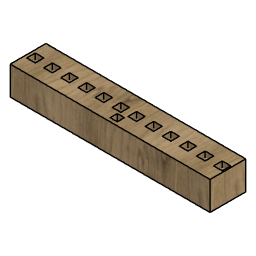
dissertation_demo2 v0 (Autodesk Fusion 360 design; units mm, degrees)
Autodesk Fusion 360 part; units mm, degrees
sketch "Sketch1" plane through (0, 0, 0) normal (0, 0, 1) x (1, 0, 0)
  line L0 (280, 50) -> (-280, 50)
  line L1 (-280, 50) -> (-280, -50)
  line L2 (-280, -50) -> (280, -50)
  line L3 (280, -50) -> (280, 50)
  line L4 (280, 50) -> (-280, -50) construction
  line L5 (-280, 50) -> (280, -50) construction
  dimension "d1" = 560
  dimension "d2" = 100
  constraint horizontal L0
  constraint perpendicular L0 L1
  constraint parallel L0 L2
  constraint parallel L1 L3
  constraint coincident L4 origin
  constraint coincident L5 origin
  measures "d1" distance of L1.end L2.end
  measures "d2" distance of L0.end L1.end
extrude "Extrude1" add sketch "Sketch1" along normal blind 50 makes body 1
sketch "Sketch2" plane through (0, 0, 50) normal (0, 0, 1) x (-1, 0, 0)
  line L0 (-280, 50) -> (-280, -50)
  line L1 (-280, -50) -> (280, -50)
  line L2 (280, -50) -> (280, 50)
  line L3 (280, 50) -> (-280, 50)
  line L4 (8, -12) -> (32, -12)
  line L5 (32, -12) -> (32, 12)
  line L6 (32, 12) -> (8, 12)
  line L7 (8, 12) -> (8, -12)
  dimension "d5" = 24
  dimension "d6" = 24
  constraint horizontal L4
  constraint vertical L5
  constraint horizontal L6
  constraint vertical L7
  measures "d5" distance of L4.start L4.end
  measures "d6" distance of L4.start L6.end
extrude "Extrude2" cut sketch "Sketch2" against normal blind 175 contours L4 L5 L6 L7 bodies 1
sketch "Sketch3" plane through (0, 0, 0) normal (0, 0, -1) x (1, 0, 0)
  line L0 (-8, -12) -> (-32, -12)
  line L1 (-32, -12) -> (-32, 12)
  line L2 (-32, 12) -> (-8, 12)
  line L3 (-8, 12) -> (-8, -12)
  line L4 (280, -50) -> (280, 50)
  line L5 (280, 50) -> (-280, 50)
  line L6 (-280, 50) -> (-280, -50)
  line L7 (-280, -50) -> (280, -50)
  line L8 (-275, 145) -> (275, 145)
  line L9 (275, 145) -> (275, -145)
  line L10 (275, -145) -> (-275, -145)
  line L11 (-275, -145) -> (-275, 145)
  line L12 (-275, 145) -> (275, -145) construction
  line L13 (275, 145) -> (-275, -145) construction
  dimension "d9" = 550
  dimension "d10" = 290
  constraint horizontal L8
  constraint perpendicular L8 L9
  constraint parallel L8 L10
  constraint parallel L9 L11
  constraint coincident L12 origin
  constraint coincident L13 origin
  measures "d9" distance of L9.end L10.end
  measures "d10" distance of L8.end L9.end
extrude "Extrude3" cut sketch "Sketch3" along normal blind 5 contours L7 L9 L10 L11 | L5 L7 L9 L11 | L5 L8 L9 L11 bodies 1
sketch "Sketch4" plane through (0, 0, 50) normal (0, 0, 1) x (-1, 0, 0)
  line L0 (32, -12) -> (8, -12)
  line L1 (8, -12) -> (8, 12)
  line L2 (8, 12) -> (32, 12)
  line L3 (32, 12) -> (32, -12)
  line L4 (-280, 50) -> (-280, -50)
  line L5 (-280, -50) -> (280, -50)
  line L6 (280, -50) -> (280, 50)
  line L7 (280, 50) -> (-280, 50)
sketch "Sketch5" plane through (0, 0, 50) normal (0, 0, 1) x (1, 0, 0)
  line L0 (36, 12) -> (12, 12)
  line L1 (12, 12) -> (12, -12)
  line L2 (12, -12) -> (36, -12)
  line L3 (36, -12) -> (36, 12)
  line L4 (36, 12) -> (12, -12) construction
  line L5 (12, 12) -> (36, -12) construction
  point P0 (24, 0)
  dimension "d13" = 24
  dimension "d14" = 24
  constraint horizontal L0
  constraint perpendicular L0 L1
  constraint parallel L0 L2
  constraint parallel L1 L3
  constraint coincident L4 P0
  constraint coincident L5 P0
  measures "d13" distance of L1.end L2.end
  measures "d14" distance of L0.end L1.end
extrude "Extrude4" cut sketch "Sketch5" against normal blind 30 bodies 1
sketch "Sketch6" plane through (0, 0, 0) normal (0, 0, 1) x (1, 0, 0)
  line L0 (-275, -45) -> (275, -45)
  line L1 (275, -45) -> (275, 45)
  line L2 (275, 45) -> (-275, 45)
  line L3 (-275, 45) -> (-275, -45)
  line L4 (-275, -45) -> (275, 45) construction
  line L5 (275, -45) -> (-275, 45) construction
  dimension "d17" = 550
  dimension "d18" = 90
  constraint horizontal L0
  constraint perpendicular L0 L1
  constraint parallel L0 L2
  constraint parallel L1 L3
  constraint coincident L4 origin
  constraint coincident L5 origin
  measures "d17" distance of L1.end L2.end
  measures "d18" distance of L0.end L1.end
extrude "Extrude5" cut sketch "Sketch6" along normal blind 30 bodies 1
sketch "Sketch7" plane through (0, 0, 50) normal (0, 0, 1) x (1, 0, 0)
  line L0 (-80, 12) -> (-56, 12)
  line L1 (-56, 12) -> (-56, -12)
  line L2 (-56, -12) -> (-80, -12)
  line L3 (-80, -12) -> (-80, 12)
  line L4 (-80, 12) -> (-56, -12) construction
  line L5 (-56, 12) -> (-80, -12) construction
  line L6 (-104, 12) -> (-128, -12) construction
  line L7 (-128, 12) -> (-104, 12)
  line L8 (-128, -12) -> (-128, 12)
  line L9 (-128, 12) -> (-104, -12) construction
  line L10 (-104, -12) -> (-128, -12)
  line L11 (-104, 12) -> (-104, -12)
  line L12 (-152, 12) -> (-176, -12) construction
  line L13 (-176, 12) -> (-152, 12)
  line L14 (-176, -12) -> (-176, 12)
  line L15 (-176, 12) -> (-152, -12) construction
  line L16 (-152, -12) -> (-176, -12)
  line L17 (-152, 12) -> (-152, -12)
  line L18 (-200, 12) -> (-224, -12) construction
  line L19 (-224, 12) -> (-200, 12)
  line L20 (-224, -12) -> (-224, 12)
  line L21 (-224, 12) -> (-200, -12) construction
  line L22 (-200, -12) -> (-224, -12)
  line L23 (-200, 12) -> (-200, -12)
  line L24 (-248, 12) -> (-272, -12) construction
  line L25 (-272, 12) -> (-248, 12)
  line L26 (-272, -12) -> (-272, 12)
  line L27 (-272, 12) -> (-248, -12) construction
  line L28 (-248, -12) -> (-272, -12)
  line L29 (-248, 12) -> (-248, -12)
  point P0 (-68, 0)
  dimension "d21" = 24
  dimension "d22" = 24
  dimension "d25" = -192
  dimension "d26" = 0
  constraint horizontal L0
  constraint perpendicular L0 L1
  constraint parallel L0 L2
  constraint parallel L1 L3
  constraint coincident L4 P0
  constraint coincident L5 P0
  measures "d21" distance of L1.end L2.end
  measures "d22" distance of L0.end L1.end
extrude "Extrude6" cut sketch "Sketch7" against normal blind 40 bodies 1
sketch "Sketch8" plane through (0, 0, 50) normal (0, 0, 1) x (-1, 0, 0)
  line L0 (224, 12) -> (224, -12)
  line L1 (224, -12) -> (200, -12)
  line L2 (200, -12) -> (200, 12)
  line L3 (200, 12) -> (224, 12)
  line L4 (176, 12) -> (176, -12)
  line L5 (176, -12) -> (152, -12)
  line L6 (152, -12) -> (152, 12)
  line L7 (152, 12) -> (176, 12)
  line L8 (272, 12) -> (272, -12)
  line L9 (272, -12) -> (248, -12)
  line L10 (248, -12) -> (248, 12)
  line L11 (248, 12) -> (272, 12)
  line L12 (128, 12) -> (128, -12)
  line L13 (128, -12) -> (104, -12)
  line L14 (104, -12) -> (104, 12)
  line L15 (104, 12) -> (128, 12)
  line L16 (56, -12) -> (56, 12)
  line L17 (56, 12) -> (80, 12)
  line L18 (80, 12) -> (80, -12)
  line L19 (80, -12) -> (56, -12)
  line L20 (-12, -12) -> (-36, -12)
  line L21 (-36, -12) -> (-36, 12)
  line L22 (-36, 12) -> (-12, 12)
  line L23 (-12, 12) -> (-12, -12)
  line L24 (32, -12) -> (8, -12)
  line L25 (8, -12) -> (8, 12)
  line L26 (8, 12) -> (32, 12)
  line L27 (32, 12) -> (32, -12)
  line L28 (-280, 50) -> (-280, -50)
  line L29 (-280, -50) -> (280, -50)
  line L30 (280, -50) -> (280, 50)
  line L31 (280, 50) -> (-280, 50)
  line L32 (-60, -12) -> (-84, -12)
  line L33 (-84, -12) -> (-84, 12)
  line L34 (-84, 12) -> (-60, 12)
  line L35 (-60, 12) -> (-60, -12)
  line L36 (-60, -12) -> (-84, 12) construction
  line L37 (-84, -12) -> (-60, 12) construction
  line L38 (-132, 12) -> (-108, 12)
  line L39 (-108, 12) -> (-108, -12)
  line L40 (-108, -12) -> (-132, -12)
  line L41 (-132, -12) -> (-108, 12) construction
  line L42 (-108, -12) -> (-132, 12) construction
  line L43 (-132, -12) -> (-132, 12)
  line L44 (-180, 12) -> (-156, 12)
  line L45 (-156, 12) -> (-156, -12)
  line L46 (-156, -12) -> (-180, -12)
  line L47 (-180, -12) -> (-156, 12) construction
  line L48 (-156, -12) -> (-180, 12) construction
  line L49 (-180, -12) -> (-180, 12)
  line L50 (-228, 12) -> (-204, 12)
  line L51 (-204, 12) -> (-204, -12)
  line L52 (-204, -12) -> (-228, -12)
  line L53 (-228, -12) -> (-204, 12) construction
  line L54 (-204, -12) -> (-228, 12) construction
  line L55 (-228, -12) -> (-228, 12)
  line L56 (-276, 12) -> (-252, 12)
  line L57 (-252, 12) -> (-252, -12)
  line L58 (-252, -12) -> (-276, -12)
  line L59 (-276, -12) -> (-252, 12) construction
  line L60 (-252, -12) -> (-276, 12) construction
  line L61 (-276, -12) -> (-276, 12)
  point P0 (-72, 0)
  point P1 (-120, 0)
  point P2 (-168, 0)
  point P3 (-216, 0)
  point P4 (-264, 0)
  dimension "d29" = 24
  dimension "d30" = 24
  dimension "d33" = -192
  dimension "d34" = 0
  constraint horizontal L32
  constraint perpendicular L32 L33
  constraint parallel L32 L34
  constraint parallel L33 L35
  constraint coincident L36 P0
  constraint coincident L37 P0
  measures "d29" distance of L33.end L34.end
  measures "d30" distance of L32.end L33.end
extrude "Extrude7" cut sketch "Sketch8" against normal blind 60 contours L32 L33 L34 L35 | L38 L39 L40 L43 | L44 L45 L46 L49 | L50 L51 L52 L55 | L56 L57 L58 L61 bodies 1
sketch "Sketch9" plane through (0, 0, 50) normal (0, 0, 1) x (-1, 0, 0)
  line L0 (-204, 12) -> (-204, -12)
  line L1 (-204, -12) -> (-228, -12)
  line L2 (-228, -12) -> (-228, 12)
  line L3 (-228, 12) -> (-204, 12)
  line L4 (-156, 12) -> (-156, -12)
  line L5 (-156, -12) -> (-180, -12)
  line L6 (-180, -12) -> (-180, 12)
  line L7 (-180, 12) -> (-156, 12)
  line L8 (-252, 12) -> (-252, -12)
  line L9 (-252, -12) -> (-276, -12)
  line L10 (-276, -12) -> (-276, 12)
  line L11 (-276, 12) -> (-252, 12)
  line L12 (-108, 12) -> (-108, -12)
  line L13 (-108, -12) -> (-132, -12)
  line L14 (-132, -12) -> (-132, 12)
  line L15 (-132, 12) -> (-108, 12)
  line L16 (-84, -12) -> (-84, 12)
  line L17 (-84, 12) -> (-60, 12)
  line L18 (-60, 12) -> (-60, -12)
  line L19 (-60, -12) -> (-84, -12)
  line L20 (224, 12) -> (224, -12)
  line L21 (224, -12) -> (200, -12)
  line L22 (200, -12) -> (200, 12)
  line L23 (200, 12) -> (224, 12)
  line L24 (176, 12) -> (176, -12)
  line L25 (176, -12) -> (152, -12)
  line L26 (152, -12) -> (152, 12)
  line L27 (152, 12) -> (176, 12)
  line L28 (272, 12) -> (272, -12)
  line L29 (272, -12) -> (248, -12)
  line L30 (248, -12) -> (248, 12)
  line L31 (248, 12) -> (272, 12)
  line L32 (128, 12) -> (128, -12)
  line L33 (128, -12) -> (104, -12)
  line L34 (104, -12) -> (104, 12)
  line L35 (104, 12) -> (128, 12)
  line L36 (56, -12) -> (56, 12)
  line L37 (56, 12) -> (80, 12)
  line L38 (80, 12) -> (80, -12)
  line L39 (80, -12) -> (56, -12)
  line L40 (-12, -12) -> (-36, -12)
  line L41 (-36, -12) -> (-36, 12)
  line L42 (-36, 12) -> (-12, 12)
  line L43 (-12, 12) -> (-12, -12)
  line L44 (32, -12) -> (8, -12)
  line L45 (8, -12) -> (8, 12)
  line L46 (8, 12) -> (32, 12)
  line L47 (32, 12) -> (32, -12)
  line L48 (-280, 50) -> (-280, -50)
  line L49 (-280, -50) -> (280, -50)
  line L50 (280, -50) -> (280, 50)
  line L51 (280, 50) -> (-280, 50)
  line L52 (10, 40) -> (-10, 40)
  line L53 (-10, 40) -> (-10, 20)
  line L54 (-10, 20) -> (10, 20)
  line L55 (10, 20) -> (10, 40)
  line L56 (10, 40) -> (-10, 20) construction
  line L57 (-10, 40) -> (10, 20) construction
  point P0 (0, 30)
  dimension "d37" = 20
  constraint horizontal L52
  constraint perpendicular L52 L53
  constraint parallel L52 L54
  constraint parallel L53 L55
  constraint coincident L56 P0
  constraint coincident L57 P0
  measures "d37" distance of L53.end L54.end
extrude "Extrude8" cut sketch "Sketch9" against normal blind 80 contours L52 L53 L54 L55 bodies 1
sphere "SpherePrimitive1" add diameter 24 placed x (0, 1, 0) y (0, 0, 1) z (1, 0, 0) at (0, 75, 5) separate body makes body 2
move_body "MoveFace1" bodies 2 to x (1, 0, 0) y (0, 1, 0) z (0, 0, 1) at (24, -75, 25) on bodies 2
copy_body "CopyPasteBodies1" bodies 2 makes body 3
move_body "Move1" bodies 3 to x (1, 0, 0) y (0, 1, 0) z (0, 0, 1) at (48, 0, 0)
copy_body "CopyPasteBodies2" bodies 3 makes body 4
move_body "Move2" bodies 4 to x (1, 0, 0) y (0, 1, 0) z (0, 0, 1) at (-92, 0, 0)
pattern_linear "R-Pattern1" count 6 spacing 48 along (-1, 0, 0) of bodies 4 makes body 5 at (-70.5534, 11.3769, 32.8366) makes body 6 at (-118.5534, 11.3769, 32.8366) makes body 7 at (-166.5534, 11.3769, 32.8366) makes body 8 at (-214.5534, 11.3769, 32.8366) makes body 9 at (-262.5534, 11.3769, 32.8366)
pattern_linear "R-Pattern2" count 5 spacing 48 along (1, 0, 0) of bodies 3 makes body 10 at (117.4466, 11.3769, 32.8366) makes body 11 at (165.4466, 11.3769, 32.8366) makes body 12 at (213.4466, 11.3769, 32.8366) makes body 13 at (261.4466, 11.3769, 32.8366)
move_face "OffsetFaces1" offset 30 1 faces at (-91.6667, 48.3333, 0) on bodies 1
sketch "Sketch11" plane through (-280, 0, 0) normal (-1, 0, 0) x (0, -1, 0)
  line L0 (-50, -30) -> (50, -30)
  line L1 (50, -30) -> (50, 50)
  line L2 (50, 50) -> (-50, 50)
  line L3 (-50, 50) -> (-50, -30)
  line L4 (-13.2967, 9.2725) -> (11.7033, 9.2725)
  line L5 (11.7033, 9.2725) -> (11.7033, -15.7275)
  line L6 (11.7033, -15.7275) -> (-13.2967, -15.7275)
  line L7 (-13.2967, -15.7275) -> (-13.2967, 9.2725)
  dimension "d50" = 25
  dimension "d51" = 25
  constraint horizontal L4
  constraint vertical L5
  constraint horizontal L6
  constraint vertical L7
  measures "d50" distance of L4.start L4.end
  measures "d51" distance of L4.start L6.end
extrude "Extrude9" cut sketch "Sketch11" against normal blind 20 contours L4 L5 L6 L7 bodies 1
